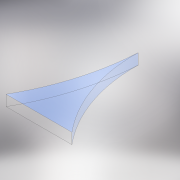
# Autodesk Inventor part: Light-Sheet
Saved by Autodesk Inventor 2020 (Build 240168000, 168)
## iProperties
Created: 2020-06-18
Part Number: Light-Sheet
Material: Generic
Document SubType Name: Modeling
Designer: MicroscopyInnovation
Density: 1 g/cm^3
Appearance: Clear - Light
Author: MicroscopyInnovation
Autodesk Inventor part; units mm, degrees
ref_plane "YZ Plane" through (0, 0, 0) normal (1, 0, 0) x (0, 1, 0)
ref_plane "XZ Plane" through (0, 0, 0) normal (0, 1, 0) x (-1, 0, 0)
ref_plane "XY Plane" through (0, 0, 0) normal (0, 0, 1) x (1, 0, 0)
sketch "Sketch1" plane through (0, 0, 0) normal (0, 1, 0) x (-1, 0, 0)
  arc A0 (1.3977, 4.7429) -> (0, 0) centre (10.7842, -0.6008) ccw
  arc A1 (0, 0) -> (-1.6641, 4.7429) centre (-7.1856, 0.1421) ccw
  line L0 (1.3977, 4.7429) -> (-1.6641, 4.7429)
  constraints: 4 point on circle, 2 centre point, 2 coincident, 2 end point
extrude "Extrusion2" add sketch "Sketch1" along normal blind 0.5
body "Solid2"
